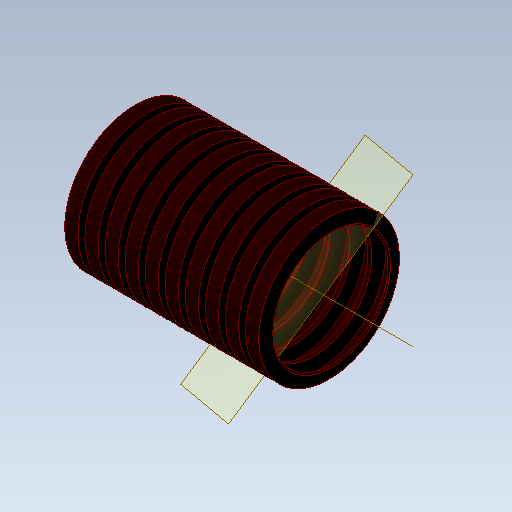
# Autodesk Inventor part: Part6
Saved by Autodesk Inventor 2020 (Build 240168000, 168)
## iProperties
Created: 2020-03-28
Part Number: Part6
Material: Generic
Document SubType Name: Modeling
Designer: Thomas Zhihao Luo
Density: 1 g/cm^3
Appearance: Default
Author: Thomas Zhihao Luo
Autodesk Inventor part; units mm, degrees
ref_plane "YZ Plane" through (0, 0, 0) normal (1, 0, 0) x (0, 1, 0)
ref_plane "XZ Plane" through (0, 0, 0) normal (0, 1, 0) x (-1, 0, 0)
ref_plane "XY Plane" through (0, 0, 0) normal (0, 0, 1) x (1, 0, 0)
ref_plane "Work Plane2" through (-4.3446, -41.309, -6.1257) normal (0, 0.7071, 0.7071) x (0.9904, -0.0979, 0.0979)
sketch "Sketch1" plane through (0, -42.2505, -5.1842) normal (0, 0.7071, 0.7071) x (-1, 0, 0)
  line L0 (-24.2607, 2.6685) -> (-23.8107, 4.6685)
  line L1 (-23.8107, 4.6685) -> (-21.9107, 4.6685)
  line L2 (-21.9107, 4.6685) -> (-21.4607, 2.6685)
  line L3 (-21.4607, 2.6685) -> (-20.7607, 2.6685)
  line L4 (-41.2554, -7.3315) -> (11.9446, -7.3315) projected
  line L5 (4.3446, -1.3315) -> (4.3446, -7.3315) projected
  line L6 (4.3446, -1.3315) -> (-17.207, 1.6821) construction
  line L7 (-24.4607, 2.9185) -> (-24.0107, 4.9185)
  line L8 (-24.0107, 4.9185) -> (-21.7107, 4.9185)
  line L9 (-21.7107, 4.9185) -> (-21.2607, 2.9185)
  line L10 (-21.2607, 2.9185) -> (-20.9867, 2.9185)
  line L11 (-20.9867, 2.9185) -> (-20.7607, 2.6685)
  line L12 (-24.4607, 2.9185) -> (-24.2607, 2.6685)
  line L13 (4.3446, -1.3315) -> (-33.6554, 3.9822) projected
  point P0 (0, -26.2099)
  point P1 (4.3446, -5.8683)
  dimension "d0" = 0.45
  dimension "d1" = 3.5
  dimension "d2" = 0.7
  dimension "d3" = 1.9
  dimension "d13" = 2
  dimension "d15" = 0.25
  dimension "d16" = 0.25
  dimension "d17" = 10
  dimension "d18" = 0.226
  constraints: 22 end point, 2 horizontal, 2 point on line, 1 equal length, 4 other
  measures "d0" horizontal distance of L1.end L2.end
  measures "d1" distance of L0.start L3.end
  measures "d2" distance of L2.end L3.end
  measures "d3" distance of L0.end L1.end
  measures "d13" distance from line of L1 L0.start
  measures "d15" distance between parallel lines of L0 L7
  measures "d16" vertical distance of L0.start L7.start
  measures "d17" distance from line of L4 L0.start
  measures "d18" horizontal distance of L3.end L10.end
revolve "Revolution1" add sketch "Sketch1" angle 360 about axis through (36.1554, -37.0663, -10.3683) along (-1, 0, 0)
pattern_linear "Rectangular Pattern2" count 10 spacing 3.5 along (-1, 0, 0) of "Revolution1"
body "Solid1"
